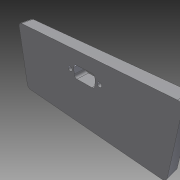
# Autodesk Inventor part: back cover
Saved by Autodesk Inventor 2012 (Build 160160000, 160)
## iProperties
Created: 2017-04-27
Part Number: back cover
Material: Default
Document SubType Name: Modeling
Designer: Brandon
Density: 1 g/cm^3
Author: Brandon
Autodesk Inventor part; units mm, degrees
ref_plane "YZ Plane" through (0, 0, 0) normal (1, 0, 0) x (0, 1, 0)
ref_plane "XZ Plane" through (0, 0, 0) normal (0, 1, 0) x (-1, 0, 0)
ref_plane "XY Plane" through (0, 0, 0) normal (0, 0, 1) x (1, 0, 0)
sketch "Sketch1" plane through (0, 0, 0) normal (0, 0, 1) x (1, 0, 0)
  line L0 (-64.5, 27.565) -> (64.5, 27.565)
  line L1 (64.5, 27.565) -> (64.5, -27.565)
  line L2 (64.5, -27.565) -> (-64.5, -27.565)
  line L3 (-64.5, -27.565) -> (-64.5, 27.565)
  point P0 (0, 0)
  dimension "d0" = 129
  dimension "d1" = 55.13
  dimension "d2" = 64.5
  dimension "d3" = 27.565
  constraints: 8 end point, 2 parallel, 1 horizontal, 1 perpendicular
  measures "d0" distance of L1.end L2.end
  measures "d1" distance of L0.end L1.end
  measures "d2" distance from line of point (0, 0) L3
  measures "d3" distance from line of L0 point (0, 0)
extrude "Extrusion1" add sketch "Sketch1" along normal blind 10.0076
fillet "Fillet1" radius 3.175 3 edges at (64.5, 27.565, 5.0038) (64.5, -27.565, 5.0038) (-64.5, -27.565, 5.0038)
fillet "Fillet2" radius 3.175 1 edges at (-64.5, 27.565, 5.0038)
sketch "Sketch5" plane through (0, 0, 10.0076) normal (0, 0, 1) x (1, 0, 0)
  line L0 (-8.885, 6.252) -> (9.115, 6.252) projected
  line L1 (9.115, 6.252) -> (9.115, 18.802) projected
  line L2 (9.115, 18.802) -> (-8.885, 18.802) projected
  line L3 (-8.885, 18.802) -> (-8.885, 6.252) projected
  circle A0 centre (-12.38, 12.527) radius 1.7859 projected
  circle A1 centre (12.61, 12.527) radius 1.7859 projected
  circle A2 centre (26.495, 9.117) radius 6.731 projected
  line L4 (2.175, 8.737) -> (14.175, 8.737) projected
  line L5 (14.175, 8.737) -> (14.175, 16.737) projected
  line L6 (14.175, 16.737) -> (2.175, 16.737) projected
  line L7 (2.175, 16.737) -> (2.175, 8.737) projected
  line L8 (2.175, 13.737) -> (2.175, 8.737) projected
  line L9 (2.175, 8.737) -> (14.175, 8.737) projected
  line L10 (14.175, 8.737) -> (14.175, 13.737) projected
  line L11 (14.175, 13.737) -> (2.175, 13.737) projected
  line L12 (47.045, 8.237) -> (63.045, 8.237) projected
  line L13 (63.045, 8.237) -> (63.045, 16.737) projected
  line L14 (63.045, 16.737) -> (47.045, 16.737) projected
  line L15 (47.045, 16.737) -> (47.045, 8.237) projected
  arc A3 (-8.885, 9.527) -> (-6.885, 7.527) centre (-6.885, 9.527) ccw projected
  line L16 (-8.885, 15.527) -> (-8.885, 9.527) projected
  arc A4 (-6.885, 17.527) -> (-8.885, 15.527) centre (-6.885, 15.527) ccw projected
  line L17 (7.115, 17.527) -> (-6.885, 17.527) projected
  arc A5 (9.115, 15.527) -> (7.115, 17.527) centre (7.115, 15.527) ccw projected
  line L18 (9.115, 9.527) -> (9.115, 15.527) projected
  arc A6 (7.115, 7.527) -> (9.115, 9.527) centre (7.115, 9.527) ccw projected
  line L19 (-6.885, 7.527) -> (7.115, 7.527) projected
  point P0 (0, 0)
extrude "Extrusion5" cut sketch "Sketch5" against normal up to surface (10.0076 mm away) contours L3 A4 L17 A5 L6 L7 L4 A6 L19 A3 | A6 L4 L7 L11 L1 | L11 L7 L6 A5 L1 | L5 A1 | A1 L11 L5 | A1 L11 | A0 picked at (13.0371, 12.3772)
equation "\"d2\" = 0.5 * d0"
equation "\"d3\" = 0.5 * d1"
body "Solid1"
